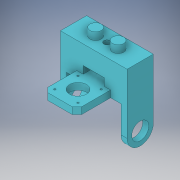
# Autodesk Inventor part: joint1_level_part_2
Saved by Autodesk Inventor 2019 (Build 230136000, 136)
## iProperties
Created: 2019-12-26
Part Number: joint1_level_part_2
Material: Пластик АБС
Document SubType Name: Modeling
Designer: Петров Иван
Density: 1.06 g/cm^3
Appearance: Серо-синий
Author: Петров Иван
Autodesk Inventor part; units mm, degrees
ref_plane "YZ Plane" through (0, 0, 0) normal (1, 0, 0) x (0, 1, 0)
ref_plane "XZ Plane" through (0, 0, 0) normal (0, 1, 0) x (-1, 0, 0)
ref_plane "XY Plane" through (0, 0, 0) normal (0, 0, 1) x (1, 0, 0)
sketch "Эскиз1" plane through (0, 0, 0) normal (1, 0, 0) x (0, 1, 0)
  line L0 (-6, -6.0208) -> (-6, 6.0208)
  arc A0 (-6, -6.0208) -> (6, -6.0208) centre (0, 0) ccw
  line L1 (6, 6.0208) -> (6, -6.0208)
  arc A1 (6, 6.0208) -> (-6, 6.0208) centre (0, 0) ccw
  circle A2 centre (0, 0) radius 17.5
  line L2 (0, 17.5) -> (80, 17.5)
  line L3 (80, 17.5) -> (80, -17.5)
  line L4 (80, -17.5) -> (0, -17.5)
  line L5 (0, -17.5) -> (0, -8.5)
  line L6 (0, 8.5) -> (0, 17.5)
  dimension "d0" = 35
  dimension "d1" = 80
  constraints: 14 end point, 6 point on circle, 3 parallel, 2 centre point, 1 coincident, 1 horizontal, 1 perpendicular, 1 vertical alignment, 2 other
  measures "d1" distance of L3.end L4.end
extrude "Выдавливание1" add sketch "Эскиз1" along normal blind 45 contours A0 L5 A2 L6 A1 L0 | A0 L1 A1 L6 A2 L5 | A2 L2 L3 L4
sketch "Эскиз2" plane through (45, 0, 0) normal (1, 0, 0) x (0, 0, -1)
  line L0 (17.5, 80) -> (-17.5, 80) projected
  line L1 (17.5, 0) -> (17.5, 80) projected
  line L2 (-17.5, 80) -> (17.5, 80)
  line L3 (17.5, 80) -> (17.5, 57)
  line L4 (17.5, 57) -> (-17.5, 57)
  line L5 (-17.5, 57) -> (-17.5, 80)
  point P0 (0, 0)
  dimension "d4" = 23
  constraints: 8 end point, 2 parallel, 1 horizontal, 1 perpendicular, 1 point on line
  measures "d4" distance of L2.end L3.end
extrude "Выдавливание2" add sketch "Эскиз2" along normal blind 22
ref_plane "РабПлоскость1" through (22.5, 0, 17.5) normal (1, 0, 0) x (0, 0, -1)
mirror "Зеркальное отражение1" about plane through (22.5, 0, 17.5) normal (1, 0, 0) of "Выдавливание2"
sketch "Эскиз3" plane through (45, 0, 0) normal (1, 0, 0) x (0, 0, -1)
  arc A0 (6.0208, -6) -> (6.0208, 6) centre (0, 0) ccw projected
  line L0 (6.0208, -6) -> (-6.0208, -6) projected
  arc A1 (-6.0208, 6) -> (-6.0208, -6) centre (0, 0) ccw projected
  line L1 (6.0208, 6) -> (-6.0208, 6) projected
  line L2 (17.5, 57) -> (-17.5, 57) projected
  line L3 (-17.5, 57) -> (-17.5, 0) projected
  arc A2 (-17.5, 0) -> (17.5, 0) centre (0, 0) ccw projected
  line L4 (17.5, 0) -> (17.5, 57) projected
sketch "Эскиз4" plane through (67, 0, 0) normal (1, 0, 0) x (0, 0, -1)
  arc A0 (6.0208, -6) -> (6.0208, 6) centre (0, 0) ccw
  line L0 (6.0208, -6) -> (-6.0208, -6)
  arc A1 (-6.0208, 6) -> (-6.0208, -6) centre (0, 0) ccw
  line L1 (6.0208, 6) -> (-6.0208, 6)
  line L2 (17.5, 37) -> (-17.5, 37)
  line L3 (-17.5, 37) -> (-17.5, 0)
  arc A2 (-17.5, 0) -> (17.5, 0) centre (0, 0) ccw
  line L4 (17.5, 0) -> (17.5, 37)
  line L5 (17.5, 0) -> (17.5, 57) projected
  line L6 (-17.5, 37) -> (17.5, 37)
  line L7 (17.5, 37) -> (17.5, 57)
  line L8 (17.5, 57) -> (-17.5, 57)
  line L9 (-17.5, 57) -> (-17.5, 37)
  constraints: 18 end point, 6 point on circle, 3 centre point, 2 parallel, 1 horizontal, 1 perpendicular
extrude "Выдавливание3" add sketch "Эскиз4" against normal blind 8
mirror "Зеркальное отражение2" about plane through (22.5, 0, 17.5) normal (1, 0, 0) of "Выдавливание3"
sketch "Эскиз5" plane through (67, 80, 17.5) normal (0, 1, 0) x (1, 0, 0)
  line L0 (-89, 35) -> (-89, 0) projected
  line L1 (-89, 35.1034) -> (-89, 0)
  line L2 (-89, 0) -> (-89, 35.1034)
  line L3 (-89, 35) -> (0, 35) projected
  line L4 (-89, 35) -> (0, 35)
  line L5 (-89, 17.5517) -> (-44.5, 17.5517)
  circle A0 centre (-44.5, 17.5517) radius 4.1
  line L6 (-44.5, 17.5517) -> (-59.5, 17.5517)
  circle A1 centre (-59.5, 17.5517) radius 7.5
  line L7 (-44.5, 17.5517) -> (-29.5, 17.5517)
  circle A2 centre (-29.5, 17.5517) radius 7.5
  point P0 (-67, 17.5)
  dimension "d9" = 8.2
  dimension "d10" = 15
  dimension "d11" = 15
  dimension "d12" = 15
  dimension "d13" = 15
  constraints: 12 end point, 3 centre point, 3 coincident, 3 collinear, 2 horizontal, 1 midpoint, 1 point on line
  measures "d9" diameter of A0
  measures "d10" distance of L6.start L6.end
  measures "d11" diameter of A1
  measures "d12" distance of L6.start L7.end
  measures "d13" diameter of A2
extrude "Выдавливание4" add sketch "Эскиз5" along normal blind 10 contours L5 A1 | L5 A1 | A2
sketch "Эскиз6" plane through (67, 80, 17.5) normal (0, 1, 0) x (1, 0, 0)
  line L0 (-89, 35) -> (-89, 0)
  line L1 (-89, 35.1034) -> (-89, 0)
  line L2 (-89, 0) -> (-89, 35.1034)
  line L3 (-89, 35) -> (0, 35)
  line L4 (-89, 35) -> (0, 35)
  line L5 (-89, 17.5517) -> (-44.5, 17.5517)
  circle A0 centre (-44.5, 17.5517) radius 4.1
  line L6 (-44.5, 17.5517) -> (-59.5, 17.5517)
  circle A1 centre (-59.5, 17.5517) radius 7.5
  line L7 (-44.5, 17.5517) -> (-29.5, 17.5517)
  circle A2 centre (-29.5, 17.5517) radius 7.5
  point P0 (-67, 17.5)
  point P1 (-67, 17.5)
  dimension "d16" = 8.2
  dimension "d17" = 15
  dimension "d18" = 15
  dimension "d19" = 15
  dimension "d20" = 15
  constraints: 16 end point, 3 centre point, 3 coincident, 3 collinear, 2 horizontal, 1 midpoint, 1 point on line
  measures "d16" diameter of A0
  measures "d17" distance of L6.start L6.end
  measures "d18" diameter of A1
  measures "d19" distance of L6.start L7.end
  measures "d20" diameter of A2
extrude "Выдавливание5" cut sketch "Эскиз6" against normal blind 35 contours A0 L7 L5 | L5 L7 A0
sketch "Эскиз7" plane through (0, 0, 17.5) normal (0, 0, 1) x (1, 0, 0)
  line L0 (18.4, 80) -> (18.4, 45) projected
  line L1 (26.6, 80) -> (26.6, 45) projected
  line L2 (0, 57) -> (0, 0) projected
  line L3 (45, 0) -> (0, 0) projected
  line L4 (45, 57) -> (45, 0) projected
  line L5 (45, 57) -> (59, 57) projected
  line L6 (67, 80) -> (67, 0) projected
  line L7 (-22, 80) -> (67, 80) projected
  line L8 (-22, 80) -> (-22, 0) projected
  line L9 (0, 57) -> (-14, 57) projected
  line L10 (18.4, 45) -> (26.6, 45) projected
  line L11 (18.4, 45) -> (8.4, 45)
  line L12 (8.4, 45) -> (8.4, 55)
  line L13 (8.4, 55) -> (36.6, 55)
  line L14 (36.6, 55) -> (36.6, 45)
  line L15 (26.6, 45) -> (36.6, 45)
  line L16 (18.4, 45) -> (26.6, 45)
  line L17 (59, 0) -> (59, 57) projected
  line L18 (67, 0) -> (59, 0) projected
  line L19 (-22, 0) -> (-14, 0) projected
  line L20 (-14, 0) -> (-14, 57) projected
  dimension "d23" = 10
  dimension "d24" = 10
  dimension "d25" = 28.2
  dimension "d26" = 10
  constraints: 12 end point, 4 perpendicular, 1 collinear, 1 horizontal, 1 point on line
  measures "d23" distance of L0.end L11.end
  measures "d24" distance of L11.end L12.end
  measures "d25" distance of L12.end L13.end
  measures "d26" distance of L1.end L14.end
extrude "Выдавливание6" cut sketch "Эскиз7" against normal blind 84.5 contours L13 L1 L10 L0 | L0 L11 L12 L13 | L13 L14 L15 L1
sketch "Эскиз8" plane through (0, 0, 17.5) normal (0, 0, 1) x (1, 0, 0)
  line L0 (8.4, 45) -> (36.6, 45) projected
  line L1 (8.4, 45) -> (0, 45)
  line L2 (0, 45) -> (0, 36)
  line L3 (0, 0) -> (0, 57) projected
  line L4 (45, -17.5) -> (45, 0) projected
  line L5 (0, 36) -> (45, 36)
  line L6 (45, 36) -> (45, -17.5)
  line L7 (45, -17.5) -> (0, -17.5)
  line L8 (0, -17.5) -> (0, 36)
  dimension "d29" = 9
  constraints: 12 end point, 2 horizontal, 2 parallel, 1 perpendicular, 1 point on line
  measures "d29" distance of L1.end L2.end
extrude "Выдавливание7" cut sketch "Эскиз8" against normal blind 85.25
sketch "Эскиз9" plane through (67, 0, 0) normal (1, 0, 0) x (0, 0, -1)
  circle A0 centre (0, 0) radius 11.4
  dimension "d32" = 22.8
  constraints: 1 centre point, 1 coincident
  measures "d32" diameter of A0
extrude "Выдавливание8" cut sketch "Эскиз9" against normal blind 144.5
sketch "Эскиз10" plane through (-22, 80, 17.5) normal (0, 0, 1) x (1, 0, 0)
  line L0 (22, -23) -> (22, -44) projected
  line L1 (67, -23) -> (67, -44) projected
  line L2 (22, -44) -> (67, -44)
  line L3 (67, -44) -> (67, -35)
  line L4 (67, -35) -> (22, -35)
  line L5 (22, -35) -> (22, -44)
  point P0 (22, -80)
  dimension "d35" = 9
  constraints: 8 end point, 2 parallel, 1 horizontal, 1 perpendicular, 1 point on line
  measures "d35" distance of L3.end L2.end
extrude "Выдавливание9" add sketch "Эскиз10" along normal blind 45
sketch "Эскиз11" plane through (67, 45, 17.5) normal (0, 1, 0) x (1, 0, 0)
  line L0 (-67, 0) -> (-67, 35) projected
  line L1 (-67, 0) -> (-44.5, 0)
  line L2 (-67, 0) -> (-58.6, 0) projected
  line L3 (-22, -45) -> (-67, -45) projected
  line L4 (-44.5, -45) -> (-44.5, -21)
  line L5 (-27, -42) -> (-23.5, -38.5)
  line L6 (-23.5, -38.5) -> (-23.5, -3.5)
  line L7 (-23.5, -3.5) -> (-27, 0)
  line L8 (-27, 0) -> (-62, 0)
  line L9 (-62, 0) -> (-65.5, -3.5)
  line L10 (-65.5, -3.5) -> (-65.5, -38.5)
  line L11 (-65.5, -38.5) -> (-62, -42)
  line L12 (-62, -42) -> (-27, -42)
  circle A0 centre (-44.5, -21) radius 11.3
  circle A1 centre (-29, -5.5) radius 1.25
  circle A2 centre (-60, -5.5) radius 1.25
  circle A3 centre (-60, -36.5) radius 1.25
  circle A4 centre (-29, -36.5) radius 1.25
  line L13 (-52.5, -48) -> (-50.5, -48)
  line L14 (-50.5, -41.8) -> (-50.5, -48)
  line L15 (-57.9172, -41.8) -> (-50.5, -41.8)
  line L16 (-65.3, -34.4172) -> (-57.9172, -41.8)
  line L17 (-65.3, -7.5828) -> (-65.3, -34.4172)
  line L18 (-57.9172, -0.2) -> (-65.3, -7.5828)
  line L19 (-31.0828, -0.2) -> (-57.9172, -0.2)
  line L20 (-23.7, -7.5828) -> (-31.0828, -0.2)
  line L21 (-23.7, -34.4172) -> (-23.7, -7.5828)
  line L22 (-31.0828, -41.8) -> (-23.7, -34.4172)
  line L23 (-38.5, -41.8) -> (-31.0828, -41.8)
  line L24 (-38.5, -41.8) -> (-38.5, -48)
  line L25 (-38.5, -48) -> (-36.5, -48)
  line L26 (-36.5, -48) -> (-36.5, -42)
  line L27 (-36.5, -42) -> (-27, -42)
  line L28 (-27, -42) -> (-23.5, -38.5)
  line L29 (-23.5, -38.5) -> (-23.5, -3.5)
  line L30 (-23.5, -3.5) -> (-27, 0)
  line L31 (-27, 0) -> (-62, 0)
  line L32 (-62, 0) -> (-65.5, -3.5)
  line L33 (-65.5, -3.5) -> (-65.5, -38.5)
  line L34 (-65.5, -38.5) -> (-62, -42)
  line L35 (-62, -42) -> (-52.5, -42)
  line L36 (-52.5, -42) -> (-52.5, -48)
  point P0 (-67, 17.5)
  dimension "d38" = 22.5
  dimension "d39" = 24
  constraints: 68 end point, 5 centre point, 1 collinear, 1 midpoint, 1 vertical
  measures "d38" distance of L0.start L1.end
  measures "d39" distance of L4.start L4.end
extrude "Выдавливание10" cut sketch "Эскиз11" against normal blind 45 contours A0 | A1 | A2 | A3 | A4
sketch "Эскиз12" plane through (67, 45, 17.5) normal (0, 1, 0) x (1, 0, 0)
  circle A0 centre (-44.5, -21) radius 11.3 projected
  circle A1 centre (-44.5, -21) radius 11.425
  point P0 (-67, 17.5)
  dimension "d42" = 22.85
  constraints: 1 centre point, 1 coincident
  measures "d42" diameter of A1
extrude "Выдавливание11" cut sketch "Эскиз12" against normal blind 45 contours A0
chamfer "Фаска1" distance 2 angle 45 4 edges at (5.75, 36, 54) (5.75, 36, 23) (36.75, 36, 23) (36.75, 36, 54)
chamfer "Фаска2" distance 6 angle 45 2 edges at (0, 40.5, 62.5) (45, 40.5, 62.5)
sketch "Эскиз13" plane through (-22, 80, 17.5) normal (0, 0, 1) x (1, 0, 0)
  line L0 (81, -80) -> (81, -23) projected
  line L1 (22, -23) -> (8, -23) projected
  line L2 (81, -44) -> (8, -44)
  line L3 (8, -44) -> (8, -23)
  line L4 (8, -23) -> (81, -23)
  line L5 (81, -23) -> (81, -44)
  line L6 (61, -44) -> (67, -44) projected
  line L7 (22, -35) -> (30.4, -35) projected
  line L8 (30.4, -25) -> (58.6, -25) projected
  line L9 (30.4, -35) -> (58.6, -35)
  line L10 (58.6, -35) -> (58.6, -25)
  line L11 (58.6, -25) -> (30.4, -25)
  line L12 (30.4, -25) -> (30.4, -35)
  point P0 (22, -80)
  dimension "d51" = 0
  constraints: 16 end point, 4 parallel, 2 horizontal, 2 perpendicular, 1 point on line
  measures "d51" distance between parallel lines of L6 L2
extrude "Выдавливание12" add sketch "Эскиз13" against normal up to surface (35 mm away)
